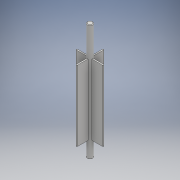
# Autodesk Inventor part: fan
Saved by Autodesk Inventor 2017 (Build 210142000, 142)
## iProperties
Created: 2017-04-22
Part Number: fan
Material: Generic
Document SubType Name: Modeling
Designer: master
Density: 1 g/cm^3
Appearance: Default
Author: master
Autodesk Inventor part; units mm, degrees
ref_plane "YZ Plane" through (0, 0, 0) normal (1, 0, 0) x (0, 1, 0)
ref_plane "XZ Plane" through (0, 0, 0) normal (0, 1, 0) x (-1, 0, 0)
sketch "Sketch1" plane through (0, 0, 0) normal (0, 0, 1) x (1, 0, 0)
  circle A0 centre (0, 0) radius 1
  dimension "d0" = 2
  constraints: 1 centre point, 1 coincident
  measures "d0" diameter of A0
extrude "Extrusion1" add sketch "Sketch1" along normal blind 40 and the other way blind 3
ref_plane "Work Plane1" through (0, 0, 29) normal (0, 0, 1) x (1, 0, 0)
sketch "Sketch2" plane through (0, 0, 29) normal (0, 0, 1) x (1, 0, 0)
  circle A0 centre (0, 0) radius 1 projected
  line L0 (-0.24, 1) -> (-0.24, 5)
  line L1 (-0.24, 5) -> (0.24, 5)
  line L2 (0.24, 5) -> (0.24, 1)
  circle A1 centre (0, 0) radius 1 projected
  line L3 (-0.24, 1) -> (-0.24, 0.957)
  line L4 (-0.24, 0.957) -> (0.24, 0.957)
  line L5 (0.24, 0.957) -> (0.24, 1)
  dimension "d5" = 4
  dimension "d6" = 0.48
  dimension "d7" = 4
  dimension "d9" = 0.24
  dimension "d10" = 5
  dimension "d11" = 5
  constraints: 12 end point, 4 perpendicular, 1 vertical
  measures "d5" distance of L0.start L0.end
  measures "d6" distance of L0.end L1.end
  measures "d7" distance of L1.end L2.end
  measures "d9" horizontal distance of L1.end point (0, 0)
  measures "d10" vertical distance of L1.end point (0, 0)
  measures "d11" distance from line of L1 point (0, 0)
extrude "Extrusion2" add sketch "Sketch2" against normal blind 26 contours L5 L4 L3 A0 | A0 L3 L0 L1 L2 L5 picked at (0.0269, 0.9702)
fillet "Fillet1" radius 0.21 2 edges at (0.24, 5, 16) (-0.24, 5, 16)
pattern_circular "Circular Pattern3" count 4 over 360 about axis through (0, 0, -10) along (0, 0, 1)
chamfer "Chamfer1" distance 0.21 angle 45 2 edges at (-1, 0, 40) (-1, 0, -3)
body "Solid1"
